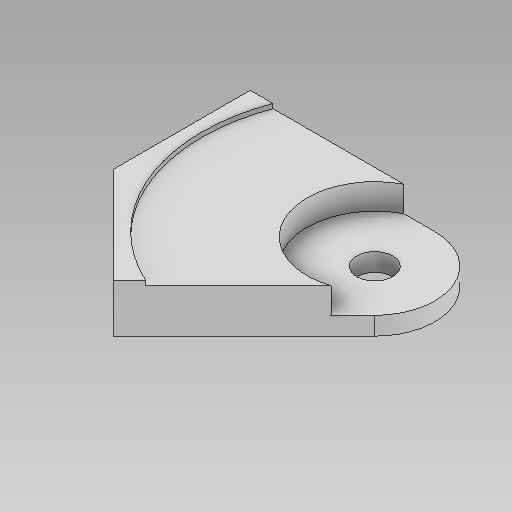
# Autodesk Inventor part: DSHR_BarCover
Saved by Autodesk Inventor 2021 (Build 250183000, 183)
## iProperties
Created: 2021-05-13
Part Number: DSHR_BarCover
Material: 一般
Document SubType Name: Modeling
Designer: kumagai
Density: 1 g/cm^3
Appearance: 既定
Author: kumagai
Autodesk Inventor part; units mm, degrees
ref_plane "YZ Plane" through (0, 0, 0) normal (1, 0, 0) x (0, 1, 0)
ref_plane "XZ Plane" through (0, 0, 0) normal (0, 1, 0) x (-1, 0, 0)
ref_plane "XY Plane" through (0, 0, 0) normal (0, 0, 1) x (1, 0, 0)
derived "DoubleSlipHR.ipt"
sketch "スケッチ1" plane through (0, 0, 0) normal (0, 1, 0) x (-1, 0, 0)
  line L0 (0, -150.5) -> (0, 150.5)
  line L1 (-115.295, 0) -> (107.7479, 0)
  line L2 (53.75, 0) -> (-53.75, 0)
  line L3 (53.75, 53.75) -> (-53.75, -53.75)
  line L4 (-0.9959, 0.9959) -> (-37.6456, 37.6456)
  line L5 (53.75, -32.2166) -> (53.75, 21.3145)
  line L6 (-53.75, -29.1125) -> (-53.75, 23.6913)
  line L7 (-63.0419, -21.9474) -> (-63.0419, 21.2839)
  line L8 (75.8846, 31.6154) -> (35.0137, 72.4863)
  line L9 (-37.2028, -70.2972) -> (-75.3835, -32.1165)
  line L10 (-50.9585, -79.0715) -> (-80.5913, -49.4386)
  line L11 (-63.0419, -19) -> (-67.2828, -19)
  line L12 (-63.0419, -17) -> (-67.2828, -17)
  line L13 (-63.0419, -9.3) -> (-67.2828, -9.3)
  line L14 (-63.0419, -6.9) -> (-67.2828, -6.9)
  line L15 (-63.0419, 6.9) -> (-67.2828, 6.9)
  line L16 (-63.0419, 9.3) -> (-67.2828, 9.3)
  line L17 (-63.0419, 17) -> (-67.2828, 17)
  line L18 (-63.0419, 19) -> (-67.2828, 19)
  line L19 (-51.5799, -78.45) -> (-56.5617, -83.4317)
  line L20 (-58.4389, -71.5911) -> (-63.4206, -76.5728)
  line L21 (-52.9942, -77.0358) -> (-57.9759, -82.0175)
  line L22 (-71.5911, -58.4389) -> (-76.5728, -63.4206)
  line L23 (-77.0358, -52.9942) -> (-82.0175, -57.9759)
  line L24 (-60.1359, -69.894) -> (-65.1177, -74.8758)
  line L25 (-69.894, -60.1359) -> (-74.8758, -65.1177)
  line L26 (-78.45, -51.5799) -> (-83.4317, -56.5617)
  line L27 (53.75, -19) -> (53.75, 19)
  line L28 (-53.75, -19) -> (-53.75, 19)
  line L29 (-53.75, -19) -> (-53.75, 19)
  line L30 (-40.315, -67.185) -> (-67.185, -40.315)
  line L31 (67.185, 40.315) -> (39.4963, 68.0037)
  arc A0 (44.528, 0) -> (-31.486, -31.486) centre (44.528, -107.5) ccw
  line L32 (44.528, -19) -> (53.75, -19)
  line L33 (53.75, -17) -> (44.528, -17)
  line L34 (-40.315, -67.185) -> (-18.051, -44.921)
  line L35 (-19.4652, -43.5068) -> (-41.7292, -65.7708)
  line L36 (44.528, 9.3) -> (53.75, 9.3)
  line L37 (53.75, 6.9) -> (33.7701, 6.9)
  line L38 (45.8701, 19) -> (67.185, 40.315)
  arc A1 (44.528, 9.3) -> (32.7459, 8.7042) centre (44.528, -107.5) ccw
  line L39 (30.4089, 6.3673) -> (32.7459, 8.7042)
  line L40 (41.0416, 17) -> (65.7708, 41.7292)
  line L41 (45.8701, 19) -> (53.75, 19)
  line L42 (53.75, 17) -> (41.0416, 17)
  line L43 (-47.1739, -60.3261) -> (-13.8318, -26.984)
  line L44 (-58.629, -48.871) -> (-28.7581, -19)
  line L45 (-53.75, -19) -> (-45.8701, -19)
  arc A2 (-29.3096, -17) -> (-38.0621, -24.9099) centre (44.528, -107.5) ccw
  line L46 (-60.3261, -47.1739) -> (-38.0621, -24.9099)
  line L47 (-17.9674, -17) -> (-29.3096, -17)
  line L48 (-41.0416, -17) -> (-53.75, -17)
  line L49 (-67.185, -40.315) -> (-45.8701, -19)
  line L50 (-65.7708, -41.7292) -> (-41.0416, -17)
  arc A3 (-44.528, 0) -> (31.486, 31.486) centre (-44.528, 107.5) ccw
  arc A4 (-44.528, 19) -> (18.051, 44.921) centre (-44.528, 107.5) ccw
  arc A5 (-44.528, 17) -> (19.4652, 43.5068) centre (-44.528, 107.5) ccw
  line L51 (-53.75, 19) -> (-44.528, 19)
  line L52 (-44.528, 17) -> (-53.75, 17)
  line L53 (18.051, 44.921) -> (40.315, 67.185)
  line L54 (19.4652, 43.5068) -> (41.7292, 65.7708)
  line L55 (28.7581, 19) -> (58.629, 48.871)
  line L56 (38.0621, 24.9099) -> (60.3261, 47.1739)
  arc A6 (29.3096, 17) -> (38.0621, 24.9099) centre (-44.528, 107.5) ccw
  line L57 (9.2419, 19) -> (48.871, 58.629)
  line L58 (3.8478, 17) -> (47.1739, 60.3261)
  line L59 (29.3096, 17) -> (3.8478, 17)
  line L60 (9.2419, 19) -> (28.7581, 19)
  line L61 (-44.528, -9.3) -> (-53.75, -9.3)
  line L62 (-33.7701, -6.9) -> (-53.75, -6.9)
  arc A7 (-44.528, -9.3) -> (-32.7459, -8.7042) centre (-44.528, 107.5) ccw
  line L63 (-19.9701, 6.9) -> (-53.75, 6.9)
  line L64 (-53.75, 9.3) -> (-14.7416, 9.3)
  line L65 (-32.7459, -8.7042) -> (-14.7416, 9.3)
  line L66 (-33.7701, -6.9) -> (-19.9701, 6.9)
  line L67 (-40.315, -67.185) -> (-31.1226, -55.1642)
  line L68 (-31.1226, -55.1642) -> (-55.1642, -31.1226)
  line L69 (-55.1642, -31.1226) -> (-67.185, -40.315)
  line L70 (53.75, -19) -> (38.75, -17)
  line L71 (38.75, -17) -> (38.75, 17)
  line L72 (38.75, 17) -> (53.75, 19)
  line L73 (-53.75, -19) -> (-38.75, -17)
  line L74 (-38.75, -17) -> (-38.75, 17)
  line L75 (-38.75, 17) -> (-53.75, 19)
  line L76 (67.185, 40.315) -> (55.1642, 31.1226)
  line L77 (55.1642, 31.1226) -> (31.1226, 55.1642)
  line L78 (31.1226, 55.1642) -> (40.315, 67.185)
  line L79 (53.75, -6.9) -> (39.2985, -6.9)
  line L80 (53.75, -9.3) -> (36.8985, -9.3)
  line L81 (33.5202, 6.6501) -> (33.7701, 6.9)
  line L82 (-13.3667, -26.2539) -> (-11.7173, -21.7221)
  line L83 (-17.1221, -17.1874) -> (-12.7514, -19.2255)
  line L84 (-48.871, -58.629) -> (-15.5916, -25.3497)
  line L85 (-28.7581, -19) -> (-18.9138, -19)
  line L86 (-15.5916, -25.3497) -> (-14.0979, -21.2457)
  line L87 (-18.9138, -19) -> (-14.0979, -21.2457)
  line L88 (-4.1916, -33.1553) -> (-0.6423, -36.7047)
  line L89 (-0.6423, -36.7047) -> (13.3057, -22.7567)
  line L90 (14.7199, -24.1709) -> (0.772, -38.1189)
  line L91 (-2.0565, -38.1189) -> (-5.6058, -34.5695)
  arc A8 (44.528, -19) -> (14.7199, -24.1709) centre (44.528, -107.5) ccw
  arc A9 (44.528, -17) -> (14.0463, -22.2878) centre (44.528, -107.5) ccw
  arc A10 (-6.7388, -32.9214) -> (-19.4652, -43.5068) centre (44.528, -107.5) ccw
  arc A11 (-5.6058, -34.5695) -> (-18.051, -44.921) centre (44.528, -107.5) ccw
  arc A12 (14.0463, -22.2878) -> (13.3057, -22.7567) centre (14.7199, -24.1709) ccw
  arc A13 (-4.1916, -33.1553) -> (-6.7388, -32.9214) centre (-5.6058, -34.5695) ccw
  arc A14 (-2.0565, -38.1189) -> (0.772, -38.1189) centre (-0.6423, -36.7047) ccw
  circle A15 centre (24.3985, -5.3) radius 1.1
  arc A16 (44.528, -9.3) -> (-12.964, -27.8889) centre (44.528, -107.5) ccw
  line L92 (24.3985, -5.3) -> (-11.0905, -20)
  line L93 (5.4469, -13.15) -> (8.1689, -19.7214)
  circle A17 centre (0, 0) radius 1.1
  circle A18 centre (24.3985, -5.3) radius 9.987
  circle A19 centre (0, 0) radius 14.9805
  arc A20 (-11.7173, -21.7221) -> (-12.7514, -19.2255) centre (-13.5966, -21.0381) ccw
  arc A21 (-13.8318, -26.984) -> (-13.3667, -26.2539) centre (-15.2461, -25.5698) ccw
  arc A22 (-17.1221, -17.1874) -> (-17.9674, -17) centre (-17.9674, -19) ccw
  line L94 (36.8985, -9.3) -> (36.8985, -0.1223)
  line L95 (30.4089, 6.3673) -> (36.8985, -0.1223)
  line L96 (39.2985, -6.9) -> (39.2985, -0.1223)
  line L97 (38.5955, 1.5747) -> (33.5202, 6.6501)
  arc A23 (39.2985, -0.1223) -> (38.5955, 1.5747) centre (36.8985, -0.1223) ccw
  point P0 (-13.5183, -26.6705)
  point P1 (-17.524, -17)
  point P2 (-5.3569, -31.9901)
  point P3 (13.6215, -22.441)
sketch "スケッチ2" plane through (0, 0, 0) normal (0, 1, 0) x (-1, 0, 0)
  line L0 (36.8985, -9.3) -> (36.8985, -0.1223) projected
  line L1 (30.4089, 6.3673) -> (36.8985, -0.1223) projected
  circle A0 centre (24.3985, -5.3) radius 1.1 projected
  line L2 (36.6985, -9.3) -> (36.6985, -0.2052)
  line L3 (36.6985, -0.2052) -> (30.2675, 6.2258)
  line L4 (53.75, -9.3) -> (36.8985, -9.3) projected
  line L5 (30.4089, 6.3673) -> (32.7459, 8.7042) projected
  line L6 (30.2675, 6.2258) -> (21.5701, -2.4716)
  line L7 (36.6985, -9.3) -> (24.3985, -9.3)
  arc A1 (21.5701, -2.4716) -> (24.3985, -9.3) centre (24.3985, -5.3) ccw
  arc A2 (26.46, -9.3) -> (23.0278, -1.0138) centre (24.3985, -5.3) ccw
  arc A3 (35.1804, -9.3) -> (29.194, 5.1524) centre (24.3985, -5.3) ccw
  circle A4 centre (24.3985, -5.3) radius 1.2
  point P0 (0, 0)
  dimension "d1" = 0.2
  dimension "d4" = 4.5
  dimension "d9" = 23
  dimension "d12" = 2.4
  constraints: 8 end point, 6 point on circle, 4 centre point, 4 coincident, 4 point on line, 2 collinear, 1 tangent, 1 other
  measures "d1" distance between parallel lines of L2 L0
  measures "d4" radius of A2
  measures "d9" diameter of A3
  measures "d12" diameter of A4
extrude "押し出し1" add sketch "スケッチ2" along normal blind 1.2 contours L7 A1 L6 A2
extrude "押し出し2" add sketch "スケッチ2" along normal blind 3.2 contours L7 A3 L6 L3 L2
extrude "押し出し3" add sketch "スケッチ2" along normal blind 2.9 contours L7 A2 L6 A3
equation "\"d7\" = RailDepth"
equation "\"RailDepth\" = 3.2"
